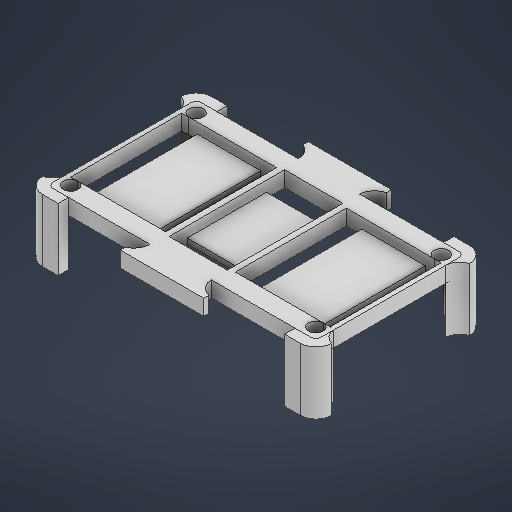
# Autodesk Inventor part: Part3
Saved by Autodesk Inventor 2026.1 (Build 301233020, 233B)
## iProperties
Created: 2025-12-24
Part Number: Part3
Material: Generic
Document SubType Name: Modeling
Designer: ferrm
Density: 1 g/cm^3
Appearance: Default
Author: ferrm
Autodesk Inventor part; units mm, degrees
ref_plane "YZ Plane" through (0, 0, 0) normal (1, 0, 0) x (0, 1, 0)
ref_plane "XZ Plane" through (0, 0, 0) normal (0, 1, 0) x (-1, 0, 0)
ref_plane "XY Plane" through (0, 0, 0) normal (0, 0, 1) x (1, 0, 0)
sketch "Sketch1" plane through (0, 0, 0) normal (0, 1, 0) x (-1, 0, 0)
  line L0 (-25.75, 13.25) -> (-25.75, -13.25)
  line L1 (-24.75, -14.25) -> (24.75, -14.25)
  line L2 (25.75, -13.25) -> (25.75, 13.25)
  line L3 (24.75, 14.25) -> (-24.75, 14.25)
  arc A0 (-25.75, -13.25) -> (-24.75, -14.25) centre (-24.75, -13.25) ccw
  arc A1 (-24.75, 14.25) -> (-25.75, 13.25) centre (-24.75, 13.25) ccw
  arc A2 (25.75, 13.25) -> (24.75, 14.25) centre (24.75, 13.25) ccw
  arc A3 (24.75, -14.25) -> (25.75, -13.25) centre (24.75, -13.25) ccw
  line L4 (24.75, -16.25) -> (-24.75, -16.25)
  arc A4 (-27.75, -13.25) -> (-24.75, -16.25) centre (-24.75, -13.25) ccw
  line L5 (-27.75, -13.25) -> (-27.75, 13.25)
  arc A5 (-24.75, 16.25) -> (-27.75, 13.25) centre (-24.75, 13.25) ccw
  line L6 (-24.75, 16.25) -> (24.75, 16.25)
  arc A6 (27.75, 13.25) -> (24.75, 16.25) centre (24.75, 13.25) ccw
  line L7 (27.75, 13.25) -> (27.75, -13.25)
  arc A7 (24.75, -16.25) -> (27.75, -13.25) centre (24.75, -13.25) ccw
  line L8 (21.75, -16.25) -> (21.75, -14.25)
  line L9 (27.75, -10.25) -> (25.75, -10.25)
  line L10 (25.75, 10.25) -> (27.75, 10.25)
  line L11 (21.75, 14.25) -> (21.75, 16.25)
  line L12 (-21.75, 14.25) -> (-21.75, 16.25)
  line L13 (-25.75, 10.25) -> (-27.75, 10.25)
  line L14 (-25.75, -10.25) -> (-27.75, -10.25)
  line L15 (-21.75, -16.25) -> (-21.75, -14.25)
  line L16 (-21.75, -14.25) -> (-17.75, -14.25)
  arc A8 (-17.75, -14.25) -> (-21.75, -16.25) centre (-15.3911, -23.9678) ccw
  line L17 (-21.75, 14.25) -> (-17.75, 14.25)
  arc A9 (-21.75, 16.25) -> (-17.75, 14.25) centre (-15.3911, 23.9678) ccw
  line L18 (-25.75, -10.25) -> (-25.75, -6.2495)
  line L19 (-25.75, 10.25) -> (-25.75, 6.25)
  arc A10 (-27.75, -10.25) -> (-25.75, -6.2495) centre (-35.468, -3.8913) ccw
  arc A11 (-25.75, 6.25) -> (-27.75, 10.25) centre (-35.4678, 3.8911) ccw
  line L20 (25.75, -10.25) -> (25.75, -6.2495)
  arc A12 (25.75, -6.2495) -> (27.75, -10.25) centre (35.468, -3.8913) ccw
  line L21 (25.75, 10.25) -> (25.75, 6.25)
  arc A13 (27.75, 10.25) -> (25.75, 6.25) centre (35.4678, 3.8911) ccw
  point P0 (0, 0)
  point P1 (-25.75, 14.25)
  point P2 (-25.75, -14.25)
  point P3 (25.75, -14.25)
  point P4 (21.75, 15.25)
  point P5 (-26.75, 10.25)
  dimension "d0" = 28.5
  dimension "d1" = 51.5
  dimension "d2" = 14.25
  dimension "d3" = 25.75
  dimension "d4" = 1
  dimension "d5" = 2
  dimension "d6" = 3
  dimension "d7" = 3
  dimension "d8" = 3
  dimension "d9" = 3
  dimension "d10" = 3
  dimension "d11" = 3
  dimension "d12" = 3
  dimension "d13" = 3
  dimension "d19" = 4
  dimension "d20" = 10
  dimension "d21" = 10
  dimension "d22" = 4
  dimension "d23" = 10
  dimension "d24" = 10
  dimension "d25" = 10
  dimension "d26" = 10
  constraints: 44 end point, 28 point on circle, 28 point on line, 14 centre point, 11 perpendicular, 8 tangent, 3 equal radius, 2 horizontal, 2 midpoint, 1 vertical, 7 other
  measures "d0" distance of point (-25.75, 14.25) point (-25.75, -14.25)
  measures "d1" distance of point (-25.75, -14.25) point (25.75, -14.25)
  measures "d2" vertical distance of point (0, 0) point (-25.75, -14.25)
  measures "d3" horizontal distance of point (0, 0) point (-25.75, -14.25)
  measures "d4" radius of A0
  measures "d5" distance between parallel lines of L1 L4
  measures "d6" distance of L4.start L8.start
  measures "d7" distance from line of L7.end L9
  measures "d8" distance of L7.start L10.end
  measures "d9" horizontal distance of L6.end point (21.75, 15.25)
  measures "d10" distance of L6.start L12.end
  measures "d11" vertical distance of L5.end point (-26.75, 10.25)
  measures "d12" distance from line of L0.end L14
  measures "d13" distance of L15.start L4.end
  measures "d19" distance of L15.end L16.end
  measures "d20" radius of A8
  measures "d21" radius of A9
  measures "d22" distance of L13.start L19.end
  measures "d23" radius of A10
  measures "d24" radius of A11
  measures "d25" radius of A12
  measures "d26" radius of A13
extrude "Extrusion1" add sketch "Sketch1" along normal blind 3.0001 contours L0 L13 L5 A5 L6 L12 L3 A1 | L0 A11 L13 | L12 A9 L3 | L0 L14 A10 | L14 L0 A0 L1 L15 L4 A4 L5 | L11 L6 A6 L7 L10 L2 A2 L3 | L15 L1 A8 | L8 L1 A3 L2 L9 L7 A7 L4 | L10 A13 L2 | L9 L2 A12
sketch "Sketch2" plane through (0, 0, 0) normal (0, -1, 0) x (1, 0, 0)
  line L0 (24.75, 14.25) -> (-24.75, 14.25) projected
  arc A0 (25.75, 13.25) -> (24.75, 14.25) centre (24.75, 13.25) ccw projected
  line L1 (-24.75, 14.25) -> (24.75, 14.25)
  line L2 (25.75, -13.25) -> (25.75, 13.25) projected
  line L3 (-24.75, -14.25) -> (24.75, -14.25) projected
  arc A1 (-25.75, -13.25) -> (-24.75, -14.25) centre (-24.75, -13.25) ccw projected
  arc A2 (24.75, -14.25) -> (25.75, -13.25) centre (24.75, -13.25) ccw projected
  line L4 (-25.75, 13.25) -> (-25.75, -13.25) projected
  arc A3 (-24.75, 14.25) -> (-25.75, 13.25) centre (-24.75, 13.25) ccw projected
  line L5 (24.75, -16.25) -> (-24.75, -16.25)
  arc A4 (-27.75, -13.25) -> (-24.75, -16.25) centre (-24.75, -13.25) ccw
  line L6 (-27.75, -13.25) -> (-27.75, 13.25)
  arc A5 (-24.75, 16.25) -> (-27.75, 13.25) centre (-24.75, 13.25) ccw
  line L7 (-24.75, 16.25) -> (24.75, 16.25)
  arc A6 (27.75, 13.25) -> (24.75, 16.25) centre (24.75, 13.25) ccw
  line L8 (27.75, 13.25) -> (27.75, -13.25)
  arc A7 (24.75, -16.25) -> (27.75, -13.25) centre (24.75, -13.25) ccw
  point P0 (0, 0)
  dimension "d16" = 2
  constraints: 10 end point, 8 point on circle, 4 centre point, 1 horizontal, 1 tangent, 7 other
  measures "d16" distance between parallel lines of L3 L5
extrude "Extrusion2" add sketch "Sketch2" against normal blind 3 contours A0 L2 A2 L3 A1 L4 A3 L0
sketch "Sketch3" plane through (0, 3, 0) normal (0, 1, 0) x (1, 0, 0)
  line L0 (6.7, 10.65) -> (24.9, 10.65)
  line L1 (24.9, 10.65) -> (24.9, -10.65)
  line L2 (24.9, -10.65) -> (6.7, -10.65)
  line L3 (6.7, -10.65) -> (6.7, 10.65)
  line L4 (-5.6, 11.1) -> (5.6, 11.1)
  line L5 (5.6, 11.1) -> (5.6, -11.1)
  line L6 (5.6, -11.1) -> (-5.6, -11.1)
  line L7 (-5.6, -11.1) -> (-5.6, 11.1)
  line L8 (17.75, 14.25) -> (-21.75, 14.25) projected
  line L9 (-21.75, -14.25) -> (17.75, -14.25) projected
  line L10 (-6.7, -10.65) -> (-24.9, -10.65)
  line L11 (-6.7, 10.65) -> (-6.7, -10.65)
  line L12 (-24.9, 10.65) -> (-6.7, 10.65)
  line L13 (-24.9, -10.65) -> (-24.9, 10.65)
  point P0 (0, 0)
  dimension "d27" = 18.2
  dimension "d28" = 21.3
  dimension "d29" = 10.65
  dimension "d30" = 6.7
  dimension "d31" = 11.2
  dimension "d32" = 22.2
  dimension "d33" = 5.6
  dimension "d34" = 11.1
  dimension "d69" = 360
  constraints: 24 end point, 4 parallel, 2 horizontal, 2 perpendicular, 17 other
  measures "d27" distance of L0.start L0.end
  measures "d28" distance of L0.end L1.end
  measures "d29" vertical distance of point (0, 0) L0.start
  measures "d30" horizontal distance of point (0, 0) L0.start
  measures "d31" distance of L5.end L6.end
  measures "d32" distance of L6.end L4.start
  measures "d33" horizontal distance of L4.start point (0, 0)
  measures "d34" distance from line of L4 point (0, 0)
extrude "Extrusion3" cut sketch "Sketch3" against normal blind 2
sketch "Sketch4" plane through (0, 3, 0) normal (0, 1, 0) x (1, 0, 0)
  line L0 (-25.75, 6.2495) -> (-25.75, 13.25) projected
  line L1 (-25.75, 12.05) -> (-23.55, 12.05)
  line L2 (-24.75, 14.25) -> (-21.75, 14.25) projected
  line L3 (-23.55, 14.25) -> (-23.55, 12.05)
  circle A0 centre (-23.55, 12.05) radius 1.4
  line L4 (17.75, 14.25) -> (24.75, 14.25) projected
  line L5 (23.55, 14.25) -> (23.55, 12.05)
  line L6 (25.75, 13.25) -> (25.75, 6.2495) projected
  line L7 (25.75, 12.05) -> (23.55, 12.05)
  line L8 (24.75, -14.25) -> (17.75, -14.25) projected
  line L9 (23.55, -14.25) -> (23.55, -12.05)
  line L10 (25.75, -6.25) -> (25.75, -13.25) projected
  line L11 (25.75, -12.05) -> (23.55, -12.05)
  line L12 (-25.75, -13.25) -> (-25.75, -6.25) projected
  line L13 (-25.75, -12.05) -> (-23.55, -12.05)
  line L14 (-21.75, -14.25) -> (-24.75, -14.25) projected
  line L15 (-23.55, -14.25) -> (-23.55, -12.05)
  point P0 (0, 0)
  dimension "d39" = 2.2
  dimension "d40" = 2.2
  dimension "d41" = 2.8
  dimension "d42" = 2.2
  dimension "d43" = 2.2
  dimension "d44" = 2.2
  dimension "d45" = 2.2
  dimension "d46" = 2.2
  dimension "d48" = 2.2
  constraints: 16 end point, 8 point on line, 3 horizontal, 3 vertical, 2 perpendicular, 1 centre point, 1 coincident
  measures "d39" distance of L1.end L3.start
  measures "d40" distance of L1.start L1.end
  measures "d41" diameter of A0
  measures "d42" distance of L7.start L5.end
  measures "d43" distance of L5.end L5.start
  measures "d44" distance of L9.end L11.start
  measures "d45" distance of L9.start L9.end
  measures "d46" distance of L13.end L13.start
  measures "d48" distance of L15.start L13.end
hole "Hole1" at (-23.55, 3, -12.05) at (23.55, 3, -12.05) at (23.55, 3, 12.05) at (-23.55, 3, 12.05) direction (0, -1, 0) diameter 2.8 end through all
sketch "Sketch5" plane through (0, 0, 0) normal (0, -1, 0) x (1, 0, 0)
  line L0 (25.75, -13.25) -> (25.75, -6.2495) projected
  arc A0 (25.75, -6.2495) -> (27.75, -10.25) centre (35.468, -3.8913) ccw projected
  line L1 (27.75, -10.25) -> (27.75, -13.25) projected
  arc A1 (24.75, -16.25) -> (27.75, -13.25) centre (24.75, -13.25) ccw projected
  line L2 (24.75, -16.25) -> (21.75, -16.25) projected
  arc A2 (21.75, -16.25) -> (17.75, -14.25) centre (15.3911, -23.9678) ccw projected
  line L3 (17.75, -14.25) -> (24.75, -14.25) projected
  arc A3 (24.75, -14.25) -> (25.75, -13.25) centre (24.75, -13.25) ccw projected
  line L4 (25.75, 6.25) -> (25.75, 13.25) projected
  arc A4 (27.75, 10.25) -> (25.75, 6.25) centre (35.4678, 3.8911) ccw projected
  line L5 (27.75, 13.25) -> (27.75, 10.25) projected
  arc A5 (27.75, 13.25) -> (24.75, 16.25) centre (24.75, 13.25) ccw projected
  arc A6 (25.75, 13.25) -> (24.75, 14.25) centre (24.75, 13.25) ccw projected
  line L6 (24.75, 14.25) -> (17.75, 14.25) projected
  arc A7 (17.75, 14.25) -> (21.75, 16.25) centre (15.3911, 23.9678) ccw projected
  line L7 (21.75, 16.25) -> (24.75, 16.25) projected
  line L8 (-21.75, 14.25) -> (-24.75, 14.25) projected
  line L9 (-21.75, 16.25) -> (-21.75, 14.25) projected
  line L10 (-24.75, 16.25) -> (-21.75, 16.25) projected
  arc A8 (-24.75, 16.25) -> (-27.75, 13.25) centre (-24.75, 13.25) ccw projected
  line L11 (-27.75, 10.25) -> (-27.75, 13.25) projected
  arc A9 (-25.75, 6.25) -> (-27.75, 10.25) centre (-35.4678, 3.8911) ccw projected
  line L12 (-25.75, 13.25) -> (-25.75, 6.25) projected
  arc A10 (-24.75, 14.25) -> (-25.75, 13.25) centre (-24.75, 13.25) ccw projected
  line L13 (-27.75, -13.25) -> (-27.75, -10.25) projected
  arc A11 (-27.75, -13.25) -> (-24.75, -16.25) centre (-24.75, -13.25) ccw projected
  line L14 (-21.75, -16.25) -> (-24.75, -16.25) projected
  line L15 (-21.75, -14.25) -> (-21.75, -16.25) projected
  line L16 (-24.75, -14.25) -> (-21.75, -14.25) projected
  arc A12 (-25.75, -13.25) -> (-24.75, -14.25) centre (-24.75, -13.25) ccw projected
  line L17 (-25.75, -6.2495) -> (-25.75, -13.25) projected
  arc A13 (-27.75, -10.25) -> (-25.75, -6.2495) centre (-35.468, -3.8913) ccw projected
  point P0 (0, 0)
extrude "Extrusion4" add sketch "Sketch5" along normal blind 9
sketch "Sketch6" plane through (0, 3, 0) normal (0, 1, 0) x (1, 0, 0)
  line L0 (17.75, 14.25) -> (-21.75, 14.25) projected
  arc A0 (-6.1051, 14.25) -> (-8, 17.039) centre (-9.1051, 14.25) ccw
  line L1 (-8, 17.039) -> (-8, 18.039)
  line L2 (-8, 18.039) -> (8, 18.039)
  line L3 (8, 18.039) -> (8, 17.039)
  arc A1 (8, 17.039) -> (5.6575, 14.25) centre (8.6543, 14.1113) ccw
  line L4 (-5.6, 11.1) -> (5.6, 11.1) projected
  line L5 (-24.5, 0) -> (24.9, 0)
  line L6 (24.9, 10.65) -> (24.9, -10.65) projected
  arc A2 (-8, -17.039) -> (-6.1051, -14.25) centre (-9.1051, -14.25) ccw
  line L7 (-8, -17.039) -> (-8, -18.039)
  line L8 (-8, -18.039) -> (8, -18.039)
  line L9 (8, -18.039) -> (8, -17.039)
  arc A3 (5.6575, -14.25) -> (8, -17.039) centre (8.6543, -14.1113) ccw
  line L10 (-6.1051, -14.25) -> (5.6575, -14.25)
  line L11 (-6.1051, 14.25) -> (5.6575, 14.25)
  point P0 (0, 0)
  point P1 (0, 11.1)
  dimension "d58" = 3
  dimension "d59" = 1
  dimension "d60" = 1
  dimension "d61" = 3
  dimension "d62" = 16
  dimension "d63" = 8
  constraints: 18 end point, 8 point on circle, 8 symmetric about line, 4 centre point, 3 point on line, 2 horizontal, 2 midpoint, 2 vertical, 1 collinear, 2 other
  measures "d58" radius of A0
  measures "d59" distance of L1.start L1.end
  measures "d60" distance of L2.end L3.end
  measures "d61" radius of A1
  measures "d62" distance of L1.end L2.end
  measures "d63" horizontal distance of point (0, 11.1) L1.end
extrude "Extrusion5" add sketch "Sketch6" against normal blind 3
sketch "Sketch7" plane through (0, 1, 0) normal (0, 1, 0) x (1, 0, 0)
  line L0 (-24.9, -10.65) -> (-24.9, 10.65) projected
  line L1 (-24.9, 10.65) -> (-21.9, 10.65)
  line L2 (-23.55, 10.65) -> (-6.7, 10.65) projected
  line L3 (-21.9, 10.65) -> (-21.9, -10.65)
  line L4 (-6.7, -10.65) -> (-23.55, -10.65) projected
  line L5 (-21.9, -10.65) -> (-24.9, -10.65)
  line L6 (-24.9, 10.65) -> (-24.9, -10.65)
  line L7 (-6.7, 10.65) -> (-6.7, -10.65) projected
  line L8 (-6.7, 10.65) -> (-9.7, 10.65)
  line L9 (-9.7, 10.65) -> (-9.7, -10.65)
  line L10 (-9.7, -10.65) -> (-6.7, -10.65)
  line L11 (-6.7, 10.65) -> (-6.7, -10.65)
  line L12 (-5.6, 11.1) -> (5.6, 11.1) projected
  line L13 (-5.6, 11.1) -> (-5.6, 7.6)
  line L14 (-5.6, 7.6) -> (5.6, 7.6)
  line L15 (5.6, 7.6) -> (5.6, 11.1)
  line L16 (5.6, 11.1) -> (-5.6, 11.1)
  line L17 (5.6, -11.1) -> (-5.6, -11.1) projected
  line L18 (-5.6, -11.1) -> (-5.6, -7.6)
  line L19 (-5.6, -11.1) -> (-5.6, 11.1) projected
  line L20 (-5.6, -7.6) -> (6.15, -7.6)
  line L21 (6.15, -7.6) -> (6.15, -11.1)
  line L22 (6.15, -11.1) -> (-5.6, -11.1)
  line L23 (6.7, 10.65) -> (23.55, 10.65) projected
  line L24 (6.7, 10.65) -> (9.7, 10.65)
  line L25 (9.7, 10.65) -> (9.7, -10.65)
  line L26 (23.55, -10.65) -> (6.7, -10.65) projected
  line L27 (6.7, -10.65) -> (6.7, 10.65)
  line L28 (23.55, 10.65) -> (24.9, 10.65) projected
  line L29 (24.9, 10.65) -> (21.9, 10.65)
  line L30 (21.9, 10.65) -> (21.9, -10.65)
  line L31 (24.9, 10.65) -> (24.9, -10.65) projected
  line L32 (24.9, -10.65) -> (24.9, 10.65)
  line L33 (24.9, 10.65) -> (24.9, -10.65)
  line L34 (21.9, -10.65) -> (24.9, -10.65)
  line L35 (21.9, 10.65) -> (24.9, 10.65)
  point P0 (0, 0)
  point P1 (5.875, -11.3)
  point P2 (-23.55, -10.65)
  dimension "d71" = 3
  dimension "d72" = 3
  dimension "d73" = 3.5
  dimension "d74" = 3.5
  dimension "d75" = 3
  dimension "d76" = 3
  constraints: 50 end point, 10 perpendicular, 9 point on line, 6 collinear, 2 parallel, 1 horizontal, 1 vertical
  measures "d71" distance of L0.end L1.end
  measures "d72" distance of L2.end L8.end
  measures "d73" distance of L12.start L13.end
  measures "d74" distance of L17.end L18.end
  measures "d75" distance of L23.start L24.end
  measures "d76" distance of L28.end L29.end
extrude "Extrusion6" cut sketch "Sketch7" against normal through all contours L0 L1 L3 L4 L5 | L9 L2 L7 L4 | L20 L21 L22 L17 L18 | L12 L15 L14 L13 | L23 L25 L26 L27 | L23 L28 L31 L34 L26 L30
sketch "Sketch9" plane through (0, 3.0001, 0) normal (0, 1, 0) x (1, 0, 0)
  line L0 (-24.9, 10.65) -> (-23.55, 10.65) projected
  line L1 (-24.9, 10.65) -> (-25.75, 10.65)
  line L2 (-25.75, 6.2495) -> (-25.75, 13.25) projected
  line L3 (-27.75, 13.25) -> (-27.75, 10.25) projected
  arc A0 (-25.75, 10.65) -> (-27.75, 13.25) centre (-28.1706, 10.8572) ccw
  line L4 (-25.75, 10.65) -> (-25.75, -10.65)
  line L5 (-25.75, -13.25) -> (-25.75, -6.25) projected
  line L6 (-25.75, -10.65) -> (25.7428, -10.65)
  line L7 (23.55, -10.65) -> (6.7, -10.65) projected
  line L8 (25.75, 13.25) -> (25.75, 6.2495) projected
  line L9 (25.75, 10.65) -> (-25.75, 10.65)
  arc A1 (27.75, 13.25) -> (24.75, 16.25) centre (24.75, 13.25) ccw projected
  arc A2 (27.75, 13.25) -> (25.75, 10.65) centre (28.4412, 10.6491) ccw
  arc A3 (24.75, -16.25) -> (27.75, -13.25) centre (24.75, -13.25) ccw projected
  arc A4 (25.7428, -10.65) -> (27.75, -13.25) centre (28.4291, -10.6509) ccw
  line L10 (24.75, -14.25) -> (17.75, -14.25) projected
  line L11 (-27.75, -10.25) -> (-27.75, -13.25) projected
  arc A5 (-27.75, -13.25) -> (-25.75, -10.65) centre (-28.44, -10.65) ccw
  arc A6 (-25.75, 6.2495) -> (-27.75, 10.25) centre (-35.468, 3.8913) ccw projected
  arc A7 (-27.75, -10.25) -> (-25.75, -6.25) centre (-35.4678, -3.8911) ccw projected
  arc A8 (21.75, -16.25) -> (17.75, -14.25) centre (15.3911, -23.9678) ccw projected
  line L12 (21.75, -16.25) -> (24.75, -16.25) projected
  line L13 (27.75, -13.25) -> (27.75, -10.25) projected
  arc A9 (25.75, -6.25) -> (27.75, -10.25) centre (35.4678, -3.8911) ccw projected
  line L14 (25.75, -6.25) -> (25.75, -13.25) projected
  line L15 (25.75, 13.25) -> (25.75, 6.2495) projected
  arc A10 (27.75, 10.25) -> (25.75, 6.2495) centre (35.468, 3.8913) ccw projected
  line L16 (27.75, 10.25) -> (27.75, 13.25) projected
  line L17 (24.75, 16.25) -> (21.75, 16.25) projected
  arc A11 (17.75, 14.25) -> (21.75, 16.25) centre (15.3911, 23.9678) ccw projected
  line L18 (17.75, 14.25) -> (24.75, 14.25) projected
  line L19 (21.75, 16.25) -> (21.75, 14.25)
  line L20 (21.75, -16.25) -> (21.75, -14.25)
  point P0 (0, 0)
  point P1 (25.75, -10.848)
  point P2 (-25.75, 11.0644)
  dimension "d84" = 2.4295
  dimension "d86" = 0
  constraints: 12 end point, 8 point on circle, 5 point on line, 4 centre point, 2 collinear, 2 perpendicular, 1 horizontal, 1 tangent
  measures "d84" radius of A0
  measures "d86" distance between parallel lines of L6 L7
extrude "Extrusion8" cut sketch "Sketch9" against normal through all contours L19 L18 A11 | A2 L16 A10 L8 | A8 L10 L20 | L14 A9 L13 A4 | L4 A5 L11 A7 | L2 A6 L3 A0
body "Solid1"
